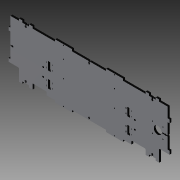
# Autodesk Inventor part: BOTTOM PLATE
Saved by Autodesk Inventor 2013 (Build 170138000, 138)
## iProperties
Created: 2014-06-21
Part Number: BOTTOM PLATE
Material: Generic
Document SubType Name: Modeling
Designer: employee
Density: 1 g/cm^3
Author: employee
Autodesk Inventor part; units mm, degrees
ref_plane "YZ Plane" through (0, 0, 0) normal (1, 0, 0) x (0, 1, 0)
ref_plane "XZ Plane" through (0, 0, 0) normal (0, 1, 0) x (-1, 0, 0)
ref_plane "XY Plane" through (0, 0, 0) normal (0, 0, 1) x (1, 0, 0)
sketch "Sketch1" plane through (0, 0, 0) normal (0, 0, 1) x (1, 0, 0)
  line L0 (-231.5, 75) -> (231.5, 75)
  line L1 (231.5, 75) -> (231.5, -75)
  line L2 (231.5, -75) -> (-231.5, -75)
  line L3 (-231.5, -75) -> (-231.5, 75)
  point P0 (0, 0)
  point P1 (0, 75)
  point P2 (-231.5, 0)
  dimension "d25" = 463
  dimension "d27" = 150
  constraints: 8 end point, 2 midpoint, 2 parallel, 1 horizontal, 1 horizontal alignment, 1 perpendicular, 1 vertical alignment
  measures "d25" distance of L0.start L0.end
  measures "d27" distance of L0.end L1.end
extrude "Extrusion1" add sketch "Sketch1" against normal blind 5.715
sketch "Sketch2" plane through (0, 0, 0) normal (0, 0, 1) x (1, 0, 0)
  line L0 (-231.5, 75) -> (231.5, 75) projected
  line L1 (-231.5, -75) -> (-231.5, 75) projected
  line L2 (231.5, -75) -> (-231.5, -75) projected
  line L3 (231.5, 75) -> (231.5, -75) projected
  line L4 (-113.25, -9) -> (113.25, -9) construction
  line L5 (113.25, -9) -> (113.25, -31) construction
  line L6 (113.25, -31) -> (-113.25, -31) construction
  line L7 (-113.25, -31) -> (-113.25, -9) construction
  line L8 (113.25, -31) -> (120.75, -31)
  line L9 (120.75, -31) -> (120.75, -55)
  line L10 (120.75, -55) -> (113.25, -55)
  line L11 (113.25, -55) -> (113.25, -31)
  line L12 (113.25, -9) -> (120.75, -9)
  line L13 (120.75, -9) -> (120.75, 15)
  line L14 (120.75, 15) -> (113.25, 15)
  line L15 (113.25, 15) -> (113.25, -9)
  line L16 (-113.25, -9) -> (-120.75, -9)
  line L17 (-120.75, -9) -> (-120.75, 15)
  line L18 (-120.75, 15) -> (-113.25, 15)
  line L19 (-113.25, 15) -> (-113.25, -9)
  line L20 (-113.25, -31) -> (-120.75, -31)
  line L21 (-120.75, -31) -> (-120.75, -55)
  line L22 (-120.75, -55) -> (-113.25, -55)
  line L23 (-113.25, -55) -> (-113.25, -31)
  line L24 (-124.5, 12) -> (-109.5, 12) construction
  line L25 (-109.5, 12) -> (-109.5, -6) construction
  line L26 (-109.5, -6) -> (-124.5, -6) construction
  line L27 (-124.5, -6) -> (-124.5, 12) construction
  line L28 (-124.5, 12) -> (-126, 12)
  line L29 (-126, 12) -> (-126, 8)
  line L30 (-126, 8) -> (-124.5, 8)
  line L31 (-124.5, 8) -> (-124.5, 12)
  line L32 (-124.5, -6) -> (-126, -6)
  line L33 (-126, -6) -> (-126, -2)
  line L34 (-126, -2) -> (-124.5, -2)
  line L35 (-124.5, -2) -> (-124.5, -6)
  line L36 (-109.5, -6) -> (-108, -6)
  line L37 (-108, -6) -> (-108, -2)
  line L38 (-108, -2) -> (-109.5, -2)
  line L39 (-109.5, -2) -> (-109.5, -6)
  line L40 (-109.5, 12) -> (-108, 12)
  line L41 (-108, 12) -> (-108, 8)
  line L42 (-108, 8) -> (-109.5, 8)
  line L43 (-109.5, 8) -> (-109.5, 12)
  line L44 (-113.25, -55) -> (-120.75, -55)
  line L45 (-120.75, -55) -> (-120.75, -31)
  line L46 (-120.75, -31) -> (-113.25, -31)
  line L47 (-113.25, -31) -> (-113.25, -55)
  line L48 (-124.5, -34) -> (-109.5, -34) construction
  line L49 (-109.5, -34) -> (-109.5, -52) construction
  line L50 (-109.5, -52) -> (-124.5, -52) construction
  line L51 (-124.5, -52) -> (-124.5, -34) construction
  line L52 (-124.5, -34) -> (-126, -34)
  line L53 (-126, -34) -> (-126, -38)
  line L54 (-126, -38) -> (-124.5, -38)
  line L55 (-124.5, -38) -> (-124.5, -34)
  line L56 (-124.5, -52) -> (-126, -52)
  line L57 (-126, -52) -> (-126, -48)
  line L58 (-126, -48) -> (-124.5, -48)
  line L59 (-124.5, -48) -> (-124.5, -52)
  line L60 (-109.5, -52) -> (-108, -52)
  line L61 (-108, -52) -> (-108, -48)
  line L62 (-108, -48) -> (-109.5, -48)
  line L63 (-109.5, -48) -> (-109.5, -52)
  line L64 (-109.5, -34) -> (-108, -34)
  line L65 (-108, -34) -> (-108, -38)
  line L66 (-108, -38) -> (-109.5, -38)
  line L67 (-109.5, -38) -> (-109.5, -34)
  line L68 (120.75, -55) -> (113.25, -55)
  line L69 (113.25, -55) -> (113.25, -31)
  line L70 (113.25, -31) -> (120.75, -31)
  line L71 (120.75, -31) -> (120.75, -55)
  line L72 (109.5, -34) -> (124.5, -34) construction
  line L73 (124.5, -34) -> (124.5, -52) construction
  line L74 (124.5, -52) -> (109.5, -52) construction
  line L75 (109.5, -52) -> (109.5, -34) construction
  line L76 (109.5, -34) -> (108, -34)
  line L77 (108, -34) -> (108, -38)
  line L78 (108, -38) -> (109.5, -38)
  line L79 (109.5, -38) -> (109.5, -34)
  line L80 (109.5, -52) -> (108, -52)
  line L81 (108, -52) -> (108, -48)
  line L82 (108, -48) -> (109.5, -48)
  line L83 (109.5, -48) -> (109.5, -52)
  line L84 (124.5, -52) -> (126, -52)
  line L85 (126, -52) -> (126, -48)
  line L86 (126, -48) -> (124.5, -48)
  line L87 (124.5, -48) -> (124.5, -52)
  line L88 (124.5, -34) -> (126, -34)
  line L89 (126, -34) -> (126, -38)
  line L90 (126, -38) -> (124.5, -38)
  line L91 (124.5, -38) -> (124.5, -34)
  line L92 (120.75, -9) -> (113.25, -9)
  line L93 (113.25, -9) -> (113.25, 15)
  line L94 (113.25, 15) -> (120.75, 15)
  line L95 (120.75, 15) -> (120.75, -9)
  line L96 (109.5, 12) -> (124.5, 12) construction
  line L97 (124.5, 12) -> (124.5, -6) construction
  line L98 (124.5, -6) -> (109.5, -6) construction
  line L99 (109.5, -6) -> (109.5, 12) construction
  line L100 (109.5, 12) -> (108, 12)
  line L101 (108, 12) -> (108, 8)
  line L102 (108, 8) -> (109.5, 8)
  line L103 (109.5, 8) -> (109.5, 12)
  line L104 (109.5, -6) -> (108, -6)
  line L105 (108, -6) -> (108, -2)
  line L106 (108, -2) -> (109.5, -2)
  line L107 (109.5, -2) -> (109.5, -6)
  line L108 (124.5, -6) -> (126, -6)
  line L109 (126, -6) -> (126, -2)
  line L110 (126, -2) -> (124.5, -2)
  line L111 (124.5, -2) -> (124.5, -6)
  line L112 (124.5, 12) -> (126, 12)
  line L113 (126, 12) -> (126, 8)
  line L114 (126, 8) -> (124.5, 8)
  line L115 (124.5, 8) -> (124.5, 12)
  point P0 (0, 0)
  point P1 (0, -9)
  point P2 (0, 75)
  point P3 (-113.25, 0)
  point P4 (-231.5, 0)
  point P5 (-126, 10)
  point P6 (-117, 12)
  point P7 (-117, 15)
  point P8 (-124.5, 3)
  point P9 (-120.75, 3)
  point P10 (-274.75, -121)
  point P11 (-126, -36)
  point P12 (-117, -34)
  point P13 (-117, -31)
  point P14 (-124.5, -43)
  point P15 (-120.75, -43)
  point P16 (-40.75, -121)
  point P17 (108, -36)
  point P18 (117, -34)
  point P19 (117, -31)
  point P20 (109.5, -43)
  point P21 (113.25, -43)
  point P22 (-40.75, -75)
  point P23 (108, 10)
  point P24 (117, 12)
  point P25 (117, 15)
  point P26 (109.5, 3)
  point P27 (113.25, 3)
  point P28 (-113.25, -20)
  dimension "d2" = 70
  dimension "d4" = 234
  dimension "d5" = 7.5
  dimension "d6" = 24
  dimension "d7" = 4
  dimension "d8" = 1.5
  dimension "d9" = 15
  dimension "d10" = 5
  dimension "d11" = 4
  dimension "d12" = 1.5
  dimension "d13" = 15
  dimension "d14" = 5
  dimension "d15" = 4
  dimension "d16" = 1.5
  dimension "d17" = 15
  dimension "d18" = 5
  dimension "d19" = 4
  dimension "d20" = 1.5
  dimension "d21" = 15
  dimension "d22" = 5
  dimension "d76" = 20
  constraints: 224 end point, 56 parallel, 30 equal length, 28 horizontal, 28 perpendicular, 23 midpoint, 5 horizontal alignment, 5 vertical alignment, 1 point on line, 2 other
  measures "d2" distance of L22.end L18.end
  measures "d4" distance between parallel lines of L9 L23
  measures "d5" distance of L21.end L22.end
  measures "d6" distance of L20.end L21.end
  measures "d7" distance of L36.end L37.end
  measures "d8" distance of L37.end L38.end
  measures "d9" distance of L24.start L24.end
  measures "d10" vertical distance of L17.end point (-126, 10)
  measures "d11" distance of L61.start L61.end
  measures "d12" distance of L61.end L63.start
  measures "d13" distance of L51.end L67.end
  measures "d14" vertical distance of L20.end point (-126, -36)
  measures "d15" distance of L85.start L85.end
  measures "d16" distance of L85.end L87.start
  measures "d17" distance of L75.end L91.end
  measures "d18" vertical distance of L5.end point (108, -36)
  measures "d19" distance of L109.start L109.end
  measures "d20" distance of L109.end L111.start
  measures "d21" distance of L99.end L115.end
  measures "d22" vertical distance of L14.end point (108, 10)
  measures "d76" vertical distance of point (0, 0) point (-113.25, -20)
extrude "Extrusion2" cut sketch "Sketch2" against normal through all keep common part
sketch "Sketch3" plane through (0, 0, 0) normal (0, 0, 1) x (1, 0, 0)
  line L0 (231.5, -75) -> (-231.5, -75) projected
  line L1 (-1.5, -66.715) -> (1.5, -66.715)
  line L2 (1.5, -66.715) -> (1.5, -75)
  line L3 (1.5, -75) -> (-1.5, -75)
  line L4 (-1.5, -75) -> (-1.5, -66.715)
  line L5 (-2.75, -68.715) -> (2.75, -68.715)
  line L6 (2.75, -68.715) -> (2.75, -70.715)
  line L7 (2.75, -70.715) -> (-2.75, -70.715)
  line L8 (-2.75, -70.715) -> (-2.75, -68.715)
  point P0 (0, 0)
  point P1 (0, -75)
  point P2 (0, -70.715)
  point P3 (0, -75)
  dimension "d31" = 3
  dimension "d32" = 6.285
  dimension "d33" = 2
  dimension "d34" = 5.5
  dimension "d35" = 2
  constraints: 16 end point, 4 midpoint, 4 parallel, 2 horizontal, 2 perpendicular, 1 vertical alignment
  measures "d31" distance of L1.start L1.end
  measures "d32" distance between parallel lines of L5 L0
  measures "d33" distance of L5.end L6.end
  measures "d34" distance of L5.start L5.end
  measures "d35" distance between parallel lines of L1 L5
extrude "Extrusion3" cut sketch "Sketch3" against normal through all
sketch "Sketch4" plane through (0, 0, 0) normal (0, 0, 1) x (1, 0, 0)
  line L0 (-1.5, -75) -> (-231.5, -75) projected
  line L1 (-1.5, -66.715) -> (1.5, -66.715) projected
  line L2 (-100, -75) -> (-50, -75)
  line L3 (-50, -75) -> (-50, -80.715)
  line L4 (-50, -80.715) -> (-100, -80.715)
  line L5 (-100, -80.715) -> (-100, -75)
  circle A0 centre (-75, -77.8575) radius 1.5
  point P0 (0, 0)
  point P1 (-75, -80.715)
  point P2 (0, -66.715)
  point P3 (-100, -77.8575)
  dimension "d39" = 5.715
  dimension "d41" = 75
  dimension "d42" = 50
  dimension "d43" = 3
  constraints: 8 end point, 3 midpoint, 2 parallel, 1 centre point, 1 horizontal, 1 horizontal alignment, 1 perpendicular, 1 point on line, 1 vertical alignment
  measures "d39" distance of L2.end L3.end
  measures "d41" horizontal distance of point (-75, -80.715) point (0, -66.715)
  measures "d42" distance of L3.end L4.end
  measures "d43" diameter of A0
extrude "Extrusion4" add sketch "Sketch4" against normal up to surface (5.715 mm away)
sketch "Sketch5" plane through (0, 0, 0) normal (0, 0, 1) x (1, 0, 0)
  line L0 (-231.5, -75) -> (-231.5, 75) projected
  line L1 (227.215, 1.5) -> (231.5, 1.5) projected
  line L2 (231.5, 1.5) -> (231.5, 35) projected
  line L3 (237.215, 35) -> (231.5, 35) projected
  line L4 (237.215, 45) -> (237.215, 35) projected
  line L5 (231.5, 45) -> (237.215, 45) projected
  line L6 (231.5, 45) -> (231.5, 83.715) projected
  line L7 (231.5, 83.715) -> (-231.5, 83.715) projected
  line L8 (-231.5, 83.715) -> (-231.5, 45) projected
  line L9 (-231.5, 45) -> (-237.215, 45) projected
  line L10 (-237.215, 45) -> (-237.215, 35) projected
  line L11 (-237.215, 35) -> (-231.5, 35) projected
  line L12 (-231.5, 35) -> (-231.5, 1.5) projected
  line L13 (-231.5, 1.5) -> (-227.215, 1.5) projected
  line L14 (-227.215, 1.5) -> (-227.215, 2.75) projected
  line L15 (-227.215, 2.75) -> (-225.215, 2.75) projected
  line L16 (-225.215, 2.75) -> (-225.215, 1.5) projected
  line L17 (-225.215, 1.5) -> (-223.215, 1.5) projected
  line L18 (-223.215, 1.5) -> (-223.215, -1.5) projected
  line L19 (-223.215, -1.5) -> (-225.215, -1.5) projected
  line L20 (-225.215, -1.5) -> (-225.215, -2.75) projected
  line L21 (-225.215, -2.75) -> (-227.215, -2.75) projected
  line L22 (-227.215, -2.75) -> (-227.215, -1.5) projected
  line L23 (-227.215, -1.5) -> (-231.5, -1.5) projected
  line L24 (-231.5, -1.5) -> (-231.5, -35) projected
  line L25 (-231.5, -35) -> (-237.215, -35) projected
  line L26 (-237.215, -35) -> (-237.215, -45) projected
  line L27 (-237.215, -45) -> (-231.5, -45) projected
  line L28 (-231.5, -45) -> (-231.5, -83.715) projected
  line L29 (-231.5, -83.715) -> (231.5, -83.715) projected
  line L30 (231.5, -83.715) -> (231.5, -45) projected
  line L31 (237.215, -45) -> (231.5, -45) projected
  line L32 (237.215, -35) -> (237.215, -45) projected
  line L33 (231.5, -35) -> (237.215, -35) projected
  line L34 (231.5, -35) -> (231.5, -1.5) projected
  line L35 (231.5, -1.5) -> (227.215, -1.5) projected
  line L36 (227.215, -1.5) -> (227.215, -2.75) projected
  line L37 (227.215, -2.75) -> (225.215, -2.75) projected
  line L38 (225.215, -2.75) -> (225.215, -1.5) projected
  line L39 (225.215, -1.5) -> (223.215, -1.5) projected
  line L40 (223.215, -1.5) -> (223.215, 1.5) projected
  line L41 (223.215, 1.5) -> (225.215, 1.5) projected
  line L42 (225.215, 1.5) -> (225.215, 2.75) projected
  line L43 (225.215, 2.75) -> (227.215, 2.75) projected
  line L44 (227.215, 2.75) -> (227.215, 1.5) projected
  circle A0 centre (0, -77.8575) radius 1.5 projected
  circle A1 centre (175, 77.8575) radius 1.5 projected
  circle A2 centre (-175, 77.8575) radius 1.5 projected
  circle A3 centre (0, 77.8575) radius 1.5 projected
  circle A4 centre (-175, -77.8575) radius 1.5 projected
  circle A5 centre (175, -77.8575) radius 1.5 projected
  line L45 (-187.5, 75) -> (-187.5, 80.715) projected
  line L46 (-197.5, 75) -> (-187.5, 75) projected
  line L47 (-197.5, 80.715) -> (-197.5, 75) projected
  line L48 (-187.5, 80.715) -> (-197.5, 80.715) projected
  line L49 (-152.5, 75) -> (-152.5, 80.715) projected
  line L50 (-162.5, 75) -> (-152.5, 75) projected
  line L51 (-162.5, 80.715) -> (-162.5, 75) projected
  line L52 (-152.5, 80.715) -> (-162.5, 80.715) projected
  line L53 (-12.5, 75) -> (-12.5, 80.715) projected
  line L54 (-22.5, 75) -> (-12.5, 75) projected
  line L55 (-22.5, 80.715) -> (-22.5, 75) projected
  line L56 (-12.5, 80.715) -> (-22.5, 80.715) projected
  line L57 (22.5, 75) -> (22.5, 80.715) projected
  line L58 (12.5, 75) -> (22.5, 75) projected
  line L59 (12.5, 80.715) -> (12.5, 75) projected
  line L60 (22.5, 80.715) -> (12.5, 80.715) projected
  line L61 (162.5, 75) -> (162.5, 80.715) projected
  line L62 (152.5, 75) -> (162.5, 75) projected
  line L63 (152.5, 80.715) -> (152.5, 75) projected
  line L64 (162.5, 80.715) -> (152.5, 80.715) projected
  line L65 (197.5, 75) -> (197.5, 80.715) projected
  line L66 (187.5, 75) -> (197.5, 75) projected
  line L67 (187.5, 80.715) -> (187.5, 75) projected
  line L68 (197.5, 80.715) -> (187.5, 80.715) projected
  line L69 (197.5, -80.715) -> (197.5, -75) projected
  line L70 (187.5, -80.715) -> (197.5, -80.715) projected
  line L71 (187.5, -75) -> (187.5, -80.715) projected
  line L72 (197.5, -75) -> (187.5, -75) projected
  line L73 (162.5, -80.715) -> (162.5, -75) projected
  line L74 (152.5, -80.715) -> (162.5, -80.715) projected
  line L75 (152.5, -75) -> (152.5, -80.715) projected
  line L76 (162.5, -75) -> (152.5, -75) projected
  line L77 (22.5, -80.715) -> (22.5, -75) projected
  line L78 (12.5, -80.715) -> (22.5, -80.715) projected
  line L79 (12.5, -75) -> (12.5, -80.715) projected
  line L80 (22.5, -75) -> (12.5, -75) projected
  line L81 (-12.5, -80.715) -> (-12.5, -75) projected
  line L82 (-22.5, -80.715) -> (-12.5, -80.715) projected
  line L83 (-22.5, -75) -> (-22.5, -80.715) projected
  line L84 (-12.5, -75) -> (-22.5, -75) projected
  line L85 (-152.5, -80.715) -> (-152.5, -75) projected
  line L86 (-162.5, -80.715) -> (-152.5, -80.715) projected
  line L87 (-162.5, -75) -> (-162.5, -80.715) projected
  line L88 (-152.5, -75) -> (-162.5, -75) projected
  line L89 (-187.5, -80.715) -> (-187.5, -75) projected
  line L90 (-197.5, -80.715) -> (-187.5, -80.715) projected
  line L91 (-197.5, -75) -> (-197.5, -80.715) projected
  line L92 (-187.5, -75) -> (-197.5, -75) projected
  point P0 (0, 0)
extrude "Extrusion5" cut sketch "Sketch5" against normal blind 5.715 contours L0 L13 L14 L15 L16 L17 L18 L19 L20 L21 L22 L23
sketch "Sketch6" plane through (0, 0, 0) normal (0, 0, 1) x (1, 0, 0)
  line L0 (-231.5, 1.5) -> (-231.5, 75) projected
  line L1 (227.215, 1.5) -> (231.5, 1.5) projected
  line L2 (231.5, 1.5) -> (231.5, 35) projected
  line L3 (237.215, 35) -> (231.5, 35) projected
  line L4 (237.215, 45) -> (237.215, 35) projected
  line L5 (231.5, 45) -> (237.215, 45) projected
  line L6 (231.5, 45) -> (231.5, 83.715) projected
  line L7 (231.5, 83.715) -> (-231.5, 83.715) projected
  line L8 (-231.5, 83.715) -> (-231.5, 45) projected
  line L9 (-231.5, 45) -> (-237.215, 45) projected
  line L10 (-237.215, 45) -> (-237.215, 35) projected
  line L11 (-237.215, 35) -> (-231.5, 35) projected
  line L12 (-231.5, 35) -> (-231.5, 1.5) projected
  line L13 (-231.5, 1.5) -> (-227.215, 1.5) projected
  line L14 (-227.215, 1.5) -> (-227.215, 2.75) projected
  line L15 (-227.215, 2.75) -> (-225.215, 2.75) projected
  line L16 (-225.215, 2.75) -> (-225.215, 1.5) projected
  line L17 (-225.215, 1.5) -> (-223.215, 1.5) projected
  line L18 (-223.215, 1.5) -> (-223.215, -1.5) projected
  line L19 (-223.215, -1.5) -> (-225.215, -1.5) projected
  line L20 (-225.215, -1.5) -> (-225.215, -2.75) projected
  line L21 (-225.215, -2.75) -> (-227.215, -2.75) projected
  line L22 (-227.215, -2.75) -> (-227.215, -1.5) projected
  line L23 (-227.215, -1.5) -> (-231.5, -1.5) projected
  line L24 (-231.5, -1.5) -> (-231.5, -35) projected
  line L25 (-231.5, -35) -> (-237.215, -35) projected
  line L26 (-237.215, -35) -> (-237.215, -45) projected
  line L27 (-237.215, -45) -> (-231.5, -45) projected
  line L28 (-231.5, -45) -> (-231.5, -83.715) projected
  line L29 (-231.5, -83.715) -> (231.5, -83.715) projected
  line L30 (231.5, -83.715) -> (231.5, -45) projected
  line L31 (237.215, -45) -> (231.5, -45) projected
  line L32 (237.215, -35) -> (237.215, -45) projected
  line L33 (231.5, -35) -> (237.215, -35) projected
  line L34 (231.5, -35) -> (231.5, -1.5) projected
  line L35 (231.5, -1.5) -> (227.215, -1.5) projected
  line L36 (227.215, -1.5) -> (227.215, -2.75) projected
  line L37 (227.215, -2.75) -> (225.215, -2.75) projected
  line L38 (225.215, -2.75) -> (225.215, -1.5) projected
  line L39 (225.215, -1.5) -> (223.215, -1.5) projected
  line L40 (223.215, -1.5) -> (223.215, 1.5) projected
  line L41 (223.215, 1.5) -> (225.215, 1.5) projected
  line L42 (225.215, 1.5) -> (225.215, 2.75) projected
  line L43 (225.215, 2.75) -> (227.215, 2.75) projected
  line L44 (227.215, 2.75) -> (227.215, 1.5) projected
  circle A0 centre (0, -77.8575) radius 1.5 projected
  circle A1 centre (175, 77.8575) radius 1.5 projected
  circle A2 centre (-175, 77.8575) radius 1.5 projected
  circle A3 centre (0, 77.8575) radius 1.5 projected
  circle A4 centre (-175, -77.8575) radius 1.5 projected
  circle A5 centre (175, -77.8575) radius 1.5 projected
  line L45 (-187.5, 75) -> (-187.5, 80.715) projected
  line L46 (-197.5, 75) -> (-187.5, 75) projected
  line L47 (-197.5, 80.715) -> (-197.5, 75) projected
  line L48 (-187.5, 80.715) -> (-197.5, 80.715) projected
  line L49 (-152.5, 75) -> (-152.5, 80.715) projected
  line L50 (-162.5, 75) -> (-152.5, 75) projected
  line L51 (-162.5, 80.715) -> (-162.5, 75) projected
  line L52 (-152.5, 80.715) -> (-162.5, 80.715) projected
  line L53 (-12.5, 75) -> (-12.5, 80.715) projected
  line L54 (-22.5, 75) -> (-12.5, 75) projected
  line L55 (-22.5, 80.715) -> (-22.5, 75) projected
  line L56 (-12.5, 80.715) -> (-22.5, 80.715) projected
  line L57 (22.5, 75) -> (22.5, 80.715) projected
  line L58 (12.5, 75) -> (22.5, 75) projected
  line L59 (12.5, 80.715) -> (12.5, 75) projected
  line L60 (22.5, 80.715) -> (12.5, 80.715) projected
  line L61 (162.5, 75) -> (162.5, 80.715) projected
  line L62 (152.5, 75) -> (162.5, 75) projected
  line L63 (152.5, 80.715) -> (152.5, 75) projected
  line L64 (162.5, 80.715) -> (152.5, 80.715) projected
  line L65 (197.5, 75) -> (197.5, 80.715) projected
  line L66 (187.5, 75) -> (197.5, 75) projected
  line L67 (187.5, 80.715) -> (187.5, 75) projected
  line L68 (197.5, 80.715) -> (187.5, 80.715) projected
  line L69 (197.5, -80.715) -> (197.5, -75) projected
  line L70 (187.5, -80.715) -> (197.5, -80.715) projected
  line L71 (187.5, -75) -> (187.5, -80.715) projected
  line L72 (197.5, -75) -> (187.5, -75) projected
  line L73 (162.5, -80.715) -> (162.5, -75) projected
  line L74 (152.5, -80.715) -> (162.5, -80.715) projected
  line L75 (152.5, -75) -> (152.5, -80.715) projected
  line L76 (162.5, -75) -> (152.5, -75) projected
  line L77 (22.5, -80.715) -> (22.5, -75) projected
  line L78 (12.5, -80.715) -> (22.5, -80.715) projected
  line L79 (12.5, -75) -> (12.5, -80.715) projected
  line L80 (22.5, -75) -> (12.5, -75) projected
  line L81 (-12.5, -80.715) -> (-12.5, -75) projected
  line L82 (-22.5, -80.715) -> (-12.5, -80.715) projected
  line L83 (-22.5, -75) -> (-22.5, -80.715) projected
  line L84 (-12.5, -75) -> (-22.5, -75) projected
  line L85 (-152.5, -80.715) -> (-152.5, -75) projected
  line L86 (-162.5, -80.715) -> (-152.5, -80.715) projected
  line L87 (-162.5, -75) -> (-162.5, -80.715) projected
  line L88 (-152.5, -75) -> (-162.5, -75) projected
  line L89 (-187.5, -80.715) -> (-187.5, -75) projected
  line L90 (-197.5, -80.715) -> (-187.5, -80.715) projected
  line L91 (-197.5, -75) -> (-197.5, -80.715) projected
  line L92 (-187.5, -75) -> (-197.5, -75) projected
  line L93 (-231.5, -45) -> (-231.5, -35)
  line L94 (-231.5, 35) -> (-231.5, 45)
  point P0 (0, 0)
  constraints: 4 end point, 1 collinear, 1 perpendicular
extrude "Extrusion6" add sketch "Sketch6" against normal blind 5.715 contours L11 L10 L9 L0 | L93 L27 L26 L25
mirror "Mirror1" about plane through (0, 0, 0) normal (0, 1, 0) of "Extrusion6", "Extrusion5", "Extrusion4", "Extrusion3"
mirror "Mirror2" about plane through (0, 0, 0) normal (1, 0, 0) of "Extrusion6", "Extrusion5", "Extrusion4", "Extrusion3", "Mirror1"
sketch "Sketch7" plane through (0, 0, 0) normal (0, 0, 1) x (1, 0, 0)
  line L0 (-231.5, -75) -> (-231.5, -45) projected
  line L1 (-100, -75) -> (-231.5, -75) projected
  line L2 (231.5, -75) -> (100, -75) projected
  line L3 (-231.5, -45) -> (-206.5, -45)
  line L4 (-206.5, -45) -> (-206.5, -75)
  line L5 (-206.5, -75) -> (-231.5, -75)
  line L6 (-231.5, -75) -> (-231.5, -45)
  line L7 (231.5, -45) -> (206.5, -45)
  line L8 (206.5, -45) -> (206.5, -75)
  line L9 (206.5, -75) -> (231.5, -75)
  line L10 (231.5, -75) -> (231.5, -45)
  point P0 (0, 0)
  dimension "d50" = 25
  constraints: 16 end point, 4 parallel, 2 horizontal, 2 perpendicular, 2 point on line, 1 collinear
  measures "d50" distance of L7.start L7.end
extrude "Extrusion7" cut sketch "Sketch7" against normal through all
sketch "Sketch8" plane through (0, 0, 0) normal (0, 0, 1) x (1, 0, 0)
  line L0 (-100, -75) -> (-206.5, -75) projected
  line L1 (-206.5, -75) -> (-196.5, -75)
  line L2 (-196.5, -75) -> (-196.5, -80.715)
  line L3 (-196.5, -80.715) -> (-206.5, -80.715)
  line L4 (-206.5, -80.715) -> (-206.5, -75)
  line L5 (-176.5, -75) -> (-166.5, -75)
  line L6 (-166.5, -75) -> (-166.5, -80.715)
  line L7 (-166.5, -80.715) -> (-176.5, -80.715)
  line L8 (-176.5, -80.715) -> (-176.5, -75)
  point P0 (0, 0)
  dimension "d53" = 20
  dimension "d55" = 10
  dimension "d56" = 5.715
  constraints: 16 end point, 4 parallel, 2 equal length, 2 horizontal, 2 perpendicular, 1 point on line
  measures "d53" distance between parallel lines of L8 L2
  measures "d55" distance of L2.end L3.end
  measures "d56" distance of L3.end L0.end
extrude "Extrusion8" add sketch "Sketch8" against normal up to surface (5.715 mm away)
sketch "Sketch10" plane through (0, 0, 0) normal (0, 0, 1) x (1, 0, 0)
  line L0 (-1.5, -66.715) -> (1.5, -66.715) projected
  line L1 (-166.5, -75) -> (-125, -75)
  line L2 (-125, -75) -> (-125, -65)
  line L3 (-125, -65) -> (-166.5, -65)
  line L4 (-166.5, -65) -> (-166.5, -75)
  point P0 (0, 0)
  point P1 (0, -66.715)
  dimension "d59" = 10
  dimension "d62" = 125
  constraints: 8 end point, 2 parallel, 1 horizontal, 1 midpoint, 1 perpendicular
  measures "d59" distance of L1.end L2.end
  measures "d62" distance from line of point (0, -66.715) L2
extrude "Extrusion9" cut sketch "Sketch10" against normal blind 5.715
sketch "Sketch11" plane through (0, 0, 0) normal (0, 0, 1) x (1, 0, 0)
  line L0 (-1.5, -66.715) -> (1.5, -66.715) projected
  line L1 (-176.5, -75) -> (-196.5, -75) projected
  line L2 (-185, -66.715) -> (-188, -66.715)
  line L3 (-188, -66.715) -> (-188, -75)
  line L4 (-188, -75) -> (-185, -75)
  line L5 (-185, -75) -> (-185, -66.715)
  line L6 (-189.25, -68.715) -> (-183.75, -68.715)
  line L7 (-183.75, -68.715) -> (-183.75, -70.715)
  line L8 (-183.75, -70.715) -> (-189.25, -70.715)
  line L9 (-189.25, -70.715) -> (-189.25, -68.715)
  point P0 (-2.75, -70.715)
  point P1 (-2.75, -68.715)
  point P2 (0, 0)
  point P3 (-186.5, -75)
  point P4 (-186.5, -75)
  point P5 (-186.5, -70.715)
  dimension "d65" = 5.5
  constraints: 16 end point, 4 midpoint, 4 parallel, 3 horizontal alignment, 2 horizontal, 2 perpendicular, 1 collinear, 1 vertical alignment
  measures "d65" distance of L6.start L6.end
extrude "Extrusion10" cut sketch "Sketch11" against normal through all
mirror "Mirror3" about plane through (0, 0, 0) normal (0, 1, 0) of "Extrusion10", "Extrusion8"
mirror "Mirror4" about plane through (0, 0, 0) normal (1, 0, 0) of "Extrusion10", "Extrusion8", "Mirror3", "Extrusion9"
fillet "Fillet1" radius 2 6 edges at (-166.5, -65, -2.8575) (-125, -65, -2.8575) (-206.5, -45, -2.8575) (206.5, -45, -2.8575) (166.5, -65, -2.8575) (125, -65, -2.8575)
sketch "Sketch12" plane through (0, 0, 0) normal (0, 0, 1) x (1, 0, 0)
  line L0 (223.215, -1.5) -> (223.215, 1.5) projected
  line L1 (223.215, -21) -> (181.215, -21) construction
  line L2 (181.215, -21) -> (181.215, 21) construction
  line L3 (181.215, 21) -> (223.215, 21) construction
  line L4 (223.215, 21) -> (223.215, -21) construction
  circle A0 centre (202.215, 0) radius 11.5
  line L5 (186.715, 15.5) -> (217.715, 15.5) construction
  line L6 (217.715, 15.5) -> (217.715, -15.5) construction
  line L7 (217.715, -15.5) -> (186.715, -15.5) construction
  line L8 (186.715, -15.5) -> (186.715, 15.5) construction
  circle A1 centre (186.715, 15.5) radius 1.5
  circle A2 centre (217.715, 15.5) radius 1.5
  circle A3 centre (186.715, -15.5) radius 1.5
  circle A4 centre (217.715, -15.5) radius 1.5
  line L9 (223.215, 1.5) -> (202.215, 1.5)
  line L10 (202.215, 1.5) -> (202.215, -1.5)
  line L11 (202.215, -1.5) -> (223.215, -1.5)
  line L12 (223.215, -1.5) -> (223.215, 1.5)
  point P0 (0, 0)
  point P1 (223.215, 0)
  point P2 (202.215, 0)
  dimension "d70" = 42
  dimension "d71" = 23
  dimension "d72" = 31
  dimension "d73" = 3
  constraints: 24 end point, 7 coincident, 5 centre point, 3 equal radius, 3 midpoint, 2 horizontal, 2 parallel, 1 perpendicular, 1 vertical alignment, 18 other
  measures "d70" distance of L1.start L1.end
  measures "d71" diameter of A0
  measures "d72" distance of L5.start L5.end
  measures "d73" diameter of A3
extrude "Extrusion11" cut sketch "Sketch12" against normal through all
sketch "Sketch13" plane through (0, 0, 0) normal (0, 0, 1) x (1, 0, 0)
  line L0 (120.75, -31) -> (113.25, -31) projected
  line L1 (113.25, -9) -> (120.75, -9) projected
  line L2 (117, -31) -> (117, -9)
  line L3 (117, -20) -> (135, -20)
  line L4 (135, -32.5) -> (135, -7.5)
  circle A0 centre (135, -32.5) radius 2.5
  circle A1 centre (135, -7.5) radius 2.5
  point P0 (0, 0)
  dimension "d78" = 5
  dimension "d79" = 25
  dimension "d82" = 135
  constraints: 6 end point, 4 midpoint, 2 centre point, 2 coincident, 2 perpendicular, 1 equal radius
  measures "d78" diameter of A0
  measures "d79" distance of L4.start L4.end
  measures "d82" distance from line of L4 point (0, 0)
extrude "Extrusion12" cut sketch "Sketch13" against normal through all
mirror "Mirror5" about plane through (0, 0, 0) normal (1, 0, 0) of "Extrusion12"
sketch "Sketch14" plane through (0, 0, 0) normal (0, 0, 1) x (1, 0, 0)
  circle A0 centre (75, -7.5) radius 2 projected
  circle A1 centre (-75, 42.5) radius 2 projected
  circle A2 centre (-75, -7.5) radius 2 projected
  circle A3 centre (75, 42.5) radius 2 projected
  line L0 (-107.5, -40) -> (107.5, -40) projected
  line L1 (107.5, -40) -> (107.5, 75) projected
  line L2 (107.5, 75) -> (-107.5, 75) projected
  line L3 (-107.5, 75) -> (-107.5, -40) projected
  point P0 (0, 0)
extrude "Extrusion13" cut sketch "Sketch14" against normal through all contours A0 | A1 | A2 | A3
sketch "Sketch15" plane through (0, 0, -5.715) normal (0, 0, -1) x (-1, 0, 0)
  line L0 (-206.5, 75) -> (-231.5, 75) projected
  line L1 (-231.5, 75) -> (-231.5, 45) projected
  line L2 (120.75, -55) -> (120.75, -31) projected
  line L3 (-231.5, 50) -> (-219, 50)
  arc A0 (-219, 50) -> (-206.5, 62.5) centre (-219, 62.5) ccw
  line L4 (-206.5, 62.5) -> (-206.5, 75)
  point P0 (0, 0)
  dimension "d85" = 25
  dimension "d86" = 12.5
  constraints: 4 end point, 3 perpendicular, 2 point on circle, 2 point on line, 2 tangent, 1 centre point
  measures "d85" distance between parallel lines of L1 L4
  measures "d86" radius of A0
extrude "Extrusion14" cut sketch "Sketch15" against normal through all
sketch "Sketch16" plane through (0, 0, -5.715) normal (0, 0, -1) x (-1, 0, 0)
  line L0 (216.5075, 63.039) -> (191.6925, 63.039) projected
  arc A0 (191.6925, 63.039) -> (186.6925, 58.039) centre (191.6925, 58.039) ccw projected
  line L1 (186.6925, 58.039) -> (186.6925, -13.639) projected
  arc A1 (186.6925, -13.639) -> (191.6925, -18.639) centre (191.6925, -13.639) ccw projected
  line L2 (191.6925, -18.639) -> (216.5075, -18.639) projected
  arc A2 (216.5075, -18.639) -> (221.5075, -13.639) centre (216.5075, -13.639) ccw projected
  line L3 (221.5075, -13.639) -> (221.5075, 58.039) projected
  arc A3 (221.5075, 58.039) -> (216.5075, 63.039) centre (216.5075, 58.039) ccw projected
  circle A4 centre (226.0075, 67.539) radius 1.5 projected
  circle A5 centre (182.1925, 67.539) radius 1.5 projected
  circle A6 centre (226.0075, -23.139) radius 1.5 projected
  arc A7 (179.1925, -23.139) -> (182.1925, -26.139) centre (182.1925, -23.139) ccw projected
  line L4 (179.1925, -23.139) -> (179.1925, 67.539) projected
  arc A8 (182.1925, 70.539) -> (179.1925, 67.539) centre (182.1925, 67.539) ccw projected
  line L5 (182.1925, 70.539) -> (226.0075, 70.539) projected
  arc A9 (229.0075, 67.539) -> (226.0075, 70.539) centre (226.0075, 67.539) ccw projected
  line L6 (229.0075, 67.539) -> (229.0075, -23.139) projected
  arc A10 (226.0075, -26.139) -> (229.0075, -23.139) centre (226.0075, -23.139) ccw projected
  line L7 (226.0075, -26.139) -> (182.1925, -26.139) projected
  circle A11 centre (182.1925, -23.139) radius 1.5 projected
  point P0 (0, 0)
extrude "Extrusion15" cut sketch "Sketch16" against normal through all contours A4 | A5 | A6 | A11
sketch "Sketch17" plane through (0, 0, -5.715) normal (0, 0, -1) x (-1, 0, 0)
  line L0 (-231.5, 35) -> (-231.5, 1.5) projected
  line L1 (-231.5, -1.5) -> (-231.5, -35) projected
  line L2 (-50, -75) -> (-1.5, -75) projected
  line L3 (-100, 75) -> (-166.5, 75) projected
  line L4 (-163, 37) -> (-161.5, 37)
  line L5 (-161.5, 37) -> (-161.5, 33)
  line L6 (-161.5, 33) -> (-163, 33)
  line L7 (-163, 33) -> (-163, 37)
  line L8 (-151.5, 37) -> (-150, 37)
  line L9 (-150, 37) -> (-150, 33)
  line L10 (-150, 33) -> (-151.5, 33)
  line L11 (-151.5, 33) -> (-151.5, 37)
  line L12 (-83.5, -56.5) -> (-83.5, -55)
  line L13 (-83.5, -55) -> (-79.5, -55)
  line L14 (-79.5, -55) -> (-79.5, -56.5)
  line L15 (-79.5, -56.5) -> (-83.5, -56.5)
  line L16 (-83.5, -45) -> (-83.5, -43.5)
  line L17 (-83.5, -43.5) -> (-79.5, -43.5)
  line L18 (-79.5, -43.5) -> (-79.5, -45)
  line L19 (-79.5, -45) -> (-83.5, -45)
  line L20 (-161.5, 35) -> (-151.5, 35)
  line L21 (-81.5, -45) -> (-81.5, -55)
  point P0 (0, 0)
  point P1 (-79.5, -55.75)
  point P2 (-79.5, -44.25)
  point P3 (-156.5, 35)
  point P4 (-81.5, -50)
  dimension "d91" = 10
  dimension "d93" = 10
  dimension "d94" = 1.5
  dimension "d95" = 4
  dimension "d96" = 40
  dimension "d97" = 75
  dimension "d98" = 25
  dimension "d99" = 150
  constraints: 36 end point, 8 midpoint, 8 parallel, 6 equal length, 4 perpendicular, 3 horizontal, 1 horizontal alignment, 1 vertical alignment
  measures "d91" distance between parallel lines of L11 L5
  measures "d93" distance between parallel lines of L19 L13
  measures "d94" distance of L16.start L16.end
  measures "d95" distance of L16.end L17.end
  measures "d96" distance from line of L3 point (-156.5, 35)
  measures "d97" distance from line of point (-156.5, 35) L0
  measures "d98" distance from line of L2 point (-81.5, -50)
  measures "d99" distance from line of point (-81.5, -50) L1
extrude "Extrusion16" cut sketch "Sketch17" against normal through all
mirror "Mirror6" about plane through (0, 0, 0) normal (1, 0, 0) of "Extrusion16"
body "Solid1"
